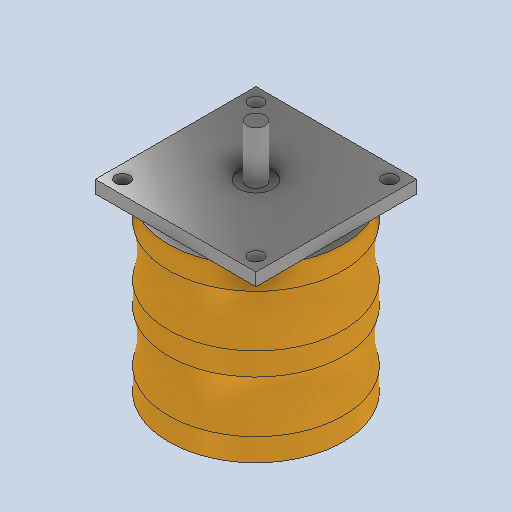
# Autodesk Inventor part: Motor
Saved by Autodesk Inventor 2023 (Build 270158000, 158)
## iProperties
Created: 2023-03-20
Part Number: Motor
Material: Steel
Document SubType Name: Sheet Metal
Designer: Mateus
Density: 7.85 g/cm^3
Sheet Metal Rule: Default_mm
Appearance: Semipolido
Mass: 1495.02 g
Surface Area: 199.529 cm^2
Volume: 190.449 cm^3
Author: Mateus
Autodesk Inventor part; units mm, degrees
ref_plane "YZ Plane" through (0, 0, 0) normal (1, 0, 0) x (0, 1, 0)
ref_plane "XZ Plane" through (0, 0, 0) normal (0, 1, 0) x (-1, 0, 0)
ref_plane "XY Plane" through (0, 0, 0) normal (0, 0, 1) x (1, 0, 0)
sketch "Esboço1" plane through (0, 0, 0) normal (0, 1, 0) x (-1, 0, 0)
  circle A0 centre (0, 0) radius 30.875
  dimension "d0" = 61.75
  constraints: 1 centre point, 1 coincident
  measures "d0" diameter of A0
extrude "Extrusão1" add sketch "Esboço1" along normal blind 60.5
sketch "Esboço2" plane through (0, 60.5, 0) normal (0, 1, 0) x (1, 0, 0)
  line L0 (-28.4, -28.4) -> (28.4, -28.4)
  line L1 (28.4, -28.4) -> (28.4, 28.4)
  line L2 (28.4, 28.4) -> (-28.4, 28.4)
  line L3 (-28.4, 28.4) -> (-28.4, -28.4)
  point P0 (0, 0)
  dimension "d3" = 56.8
  dimension "d4" = 56.8
  dimension "d5" = 28.4
  dimension "d6" = 28.4
  constraints: 8 end point, 2 parallel, 1 horizontal, 1 perpendicular
  measures "d3" distance of L2.end L0.start
  measures "d4" distance of L1.end L2.end
  measures "d5" distance from line of L2 point (0, 0)
  measures "d6" distance from line of L1 point (0, 0)
extrude "Extrusão2" add sketch "Esboço2" along normal blind 4.5
sketch "Esboço3" plane through (0, 65, 0) normal (0, 1, 0) x (1, 0, 0)
  line L0 (-28.4, -28.4) -> (28.4, -28.4) projected
  line L1 (28.4, -28.4) -> (28.4, 28.4) projected
  line L2 (-28.4, 28.4) -> (-28.4, -28.4) projected
  line L3 (28.4, 28.4) -> (-28.4, 28.4) projected
  point P0 (0, 0)
  point P1 (23.6, -23.6)
  point P2 (-23.6, -23.6)
  point P3 (-23.6, 23.6)
  point P4 (23.6, 23.6)
  dimension "d9" = 4.8
  dimension "d10" = 4.8
  dimension "d11" = 4.8
  dimension "d12" = 4.8
  dimension "d13" = 4.8
  dimension "d14" = 4.8
  dimension "d15" = 4.8
  dimension "d16" = 4.8
  measures "d9" distance from line of L0 point (23.6, -23.6)
  measures "d10" distance from line of L1 point (23.6, -23.6)
  measures "d11" distance from line of L0 point (-23.6, -23.6)
  measures "d12" distance from line of L2 point (-23.6, -23.6)
  measures "d13" distance from line of L2 point (-23.6, 23.6)
  measures "d14" distance from line of L3 point (-23.6, 23.6)
  measures "d15" distance from line of L1 point (23.6, 23.6)
  measures "d16" distance from line of L3 point (23.6, 23.6)
hole "Furo1" at (23.6, 65, 23.6) at (-23.6, 65, 23.6) at (-23.6, 65, -23.6) at (23.6, 65, -23.6) direction (0, -1, 0) diameter 5 depth 4.5
sketch "Esboço4" plane through (0, 65, 0) normal (0, 1, 0) x (1, 0, 0)
  circle A0 centre (0, 0) radius 3.25
  dimension "d24" = 6.5
  constraints: 1 centre point, 1 coincident
  measures "d24" diameter of A0
extrude "Extrusão3" add sketch "Esboço4" along normal blind 18
sketch "Esboço5" plane through (0, 65, 0) normal (0, 1, 0) x (1, 0, 0)
  circle A0 centre (0, 0) radius 6
  circle A1 centre (0, 0) radius 3.25 projected
  dimension "d27" = 12
  constraints: 1 centre point, 1 coincident
  measures "d27" diameter of A0
extrude "Extrusão4" cut sketch "Esboço5" against normal blind 0.5
sketch "Esboço6" plane through (0, 0, 0) normal (0, 0, 1) x (1, 0, 0)
  line L0 (0, 0) -> (0, 60.5)
  line L1 (-12.1122, 60.5) -> (12.1122, 60.5) projected
  line L2 (0, 60.5) -> (-30.875, 60.5)
  line L3 (-30.875, 60.5) -> (-30.875, 52.5)
  line L4 (-30.875, 0) -> (-30.875, 60.5) projected
  arc A0 (-30.875, 34.25) -> (-30.875, 52.5) centre (-65.875, 43.375) ccw
  line L5 (30.875, 0) -> (-30.875, 0) projected
  line L6 (-30.875, 0) -> (-30.875, 8)
  arc A1 (-30.875, 8) -> (-30.875, 26.25) centre (-65.875, 17.125) ccw
  line L7 (-30.875, 26.25) -> (-30.875, 34.25)
  line L8 (-30.875, 0) -> (0, 0)
  line L9 (-30.875, 60.5) -> (-66.7077, 60.5)
  line L10 (-66.7077, 60.5) -> (-66.7077, 0)
  line L11 (-66.7077, 0) -> (-30.875, 0)
  dimension "d32" = 0
  dimension "d33" = 35
  dimension "d34" = 0
  dimension "d36" = 8
  dimension "d37" = 8
  dimension "d40" = 8
  constraints: 18 end point, 4 point on circle, 3 perpendicular, 3 point on line, 2 centre point, 2 horizontal, 1 collinear, 1 equal radius, 1 midpoint, 1 vertical
  measures "d32" horizontal distance of A1.centre A0.centre
  measures "d33" horizontal distance of L4.end A0.centre
  measures "d34" distance between parallel lines of L4 L3
  measures "d36" distance of L4.end L3.end
  measures "d37" distance of L6.end L4.start
  measures "d40" distance of L7.start L7.end
revolve "Revolução1" cut sketch "Esboço6" angle 360 about axis through (0, 0, 0) along (0, 1, 0) contours L11 L10 L9 L3 L4 | L4 A1 | A0 L4
equation "\"d4\" = d3"
equation "\"d5\" = 0.5 * d3"
equation "\"d6\" = 0.5 * d4"
equation "\"d10\" = d9"
equation "\"d11\" = d10"
equation "\"d12\" = d10"
equation "\"d13\" = d12"
equation "\"d14\" = d10"
equation "\"d15\" = d9"
equation "\"d16\" = d9"
equation "\"d22\" = Espessura"
equation "\"Raio_vergadura\" = Espessura"
equation "\"Largura_alívio_de_vergadura\" = Espessura"
equation "\"Profundidade_alívio_de_vergadura\" = 0.5 * Espessura"
equation "\"Tamanho_alívio_de_dobra\" = 4 * Espessura"
equation "\"Remanescente_mínimo\" = 2 * Espessura"
equation "\"Raiodetransição\" = Raio_vergadura"
equation "\"Tamanho_de_raio_de_Jacobi\" = Raio_vergadura"
equation "\"TamanhoFolga\" = Espessura"
equation "\"Espessura\" = 0.5"
